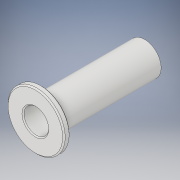
# Autodesk Inventor part: douille
Saved by Autodesk Inventor 2019 (Build 230136000, 136)
## iProperties
Created: 2018-04-17
Part Number: douille
Material: Plastique ABS
Document SubType Name: Modeling
Designer: Theo
Density: 1.06 g/cm^3
Appearance: Lisse - Blanc
Mass: 6.27305 g
Surface Area: 57.5323 cm^2
Volume: 5.91798 cm^3
Author: Theo
Autodesk Inventor part; units mm, degrees
ref_plane "YZ Plane" through (0, 0, 0) normal (1, 0, 0) x (0, 1, 0)
ref_plane "XZ Plane" through (0, 0, 0) normal (0, 1, 0) x (-1, 0, 0)
ref_plane "XY Plane" through (0, 0, 0) normal (0, 0, 1) x (1, 0, 0)
sketch "Esquisse1" plane through (0, 0, 0) normal (1, 0, 0) x (0, 1, 0)
  line L0 (13.35, -3) -> (8.5, -3)
  line L1 (8.5, -3) -> (8, -3.5)
  line L2 (8, -3.5) -> (8, -53)
  line L3 (8, -53) -> (6, -53)
  line L4 (6, -53) -> (6, -0.5)
  line L5 (6, -0.5) -> (6.5, 0)
  line L6 (6.5, 0) -> (13.225, 0)
  line L7 (13.225, 0) -> (13.85, -0.625)
  line L8 (13.85, -0.625) -> (13.85, -2.5)
  line L9 (13.85, -2.5) -> (13.35, -3)
  line L10 (0, 8.9692) -> (0, -52.1325)
  point P0 (0, 0)
  dimension "d0" = 3
  dimension "d3" = 0.5
  dimension "d4" = 0.5
  dimension "d5" = 0.5
  dimension "d6" = 0.5
  dimension "d7" = 0.625
  dimension "d8" = 0.625
  dimension "d9" = 0.5
  dimension "d10" = 0.5
  dimension "d12" = 50
  dimension "d15" = 12
  dimension "d16" = 27.7
  dimension "d17" = 16
  constraints: 22 end point, 4 vertical, 3 horizontal, 1 horizontal alignment, 1 point on line
  measures "d0" distance between parallel lines of L6 L0
  measures "d3" horizontal distance of L4.end L5.end
  measures "d4" horizontal distance of L4.end L5.end
  measures "d5" horizontal distance of L8.end L0.start
  measures "d6" horizontal distance of L8.end L0.start
  measures "d7" horizontal distance of L6.end L7.end
  measures "d8" horizontal distance of L6.end L7.end
  measures "d9" horizontal distance of L0.end L1.end
  measures "d10" horizontal distance of L0.end L1.end
  measures "d12" distance between parallel lines of L3 L0
  measures "d15" diameter of L4 L10
  measures "d16" diameter of L7.end L10
  measures "d17" diameter of L2.end L10
revolve "Révolution1" add sketch "Esquisse1" angle 360 about axis through (0, 0, 8.9692) along (0, 0, -1)
equation "\"d4\" = d3"
equation "\"d6\" = d5"
equation "\"d8\" = d7"
equation "\"d10\" = d9"
